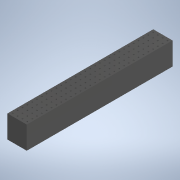
# Autodesk Inventor part: PCIconnector
Saved by Autodesk Inventor 2022 (Build 260153000, 153)
## iProperties
Created: 2021-10-06
Part Number: PCIconnector
Material: Generic
Document SubType Name: Modeling
Designer: Bowen O'Steen
Density: 1 g/cm^3
Appearance: Dark Gray
Author: Bowen O'Steen
Autodesk Inventor part; units mm, degrees
ref_plane "YZ Plane" through (0, 0, 0) normal (1, 0, 0) x (0, 1, 0)
ref_plane "XZ Plane" through (0, 0, 0) normal (0, 1, 0) x (-1, 0, 0)
ref_plane "XY Plane" through (0, 0, 0) normal (0, 0, 1) x (1, 0, 0)
sketch "Sketch1" plane through (0, 0, 0) normal (0, 1, 0) x (-1, 0, 0)
  line L0 (4, 30.15) -> (-4, 30.15)
  line L1 (-4, 30.15) -> (-4, -30.15)
  line L2 (-4, -30.15) -> (4, -30.15)
  line L3 (4, -30.15) -> (4, 30.15)
  point P0 (0, 0)
  point P1 (4, 0)
  point P2 (0, -30.15)
  dimension "d0" = 8
  dimension "d1" = 60.3
  constraints: 8 end point, 2 midpoint, 2 parallel, 1 horizontal, 1 horizontal alignment, 1 perpendicular, 1 vertical alignment
  measures "d0" distance of L1.end L2.end
  measures "d1" distance of L2.end L0.start
extrude "Extrusion1" add sketch "Sketch1" along normal blind 9.35
sketch "Sketch2" plane through (0, 9.35, 0) normal (0, 1, 0) x (1, 0, 0)
  line L0 (-3.25, 28.75) -> (-2.75, 28.75)
  line L1 (-2.75, 28.75) -> (-2.75, 29.25)
  line L2 (-2.75, 29.25) -> (-3.25, 29.25)
  line L3 (-3.25, 29.25) -> (-3.25, 28.75)
  line L4 (-4, 30.15) -> (-4, -30.15) projected
  line L5 (4, 30.15) -> (-4, 30.15) projected
  point P0 (0, 0)
  dimension "d4" = 0.5
  dimension "d5" = 0.5
  dimension "d6" = 0.75
  dimension "d7" = 0.9
  constraints: 8 end point, 2 parallel, 1 horizontal, 1 perpendicular
  measures "d4" distance of L2.end L0.start
  measures "d5" distance of L1.end L2.end
  measures "d6" distance between parallel lines of L4 L3
  measures "d7" distance between parallel lines of L5 L2
extrude "Extrusion2" cut sketch "Sketch2" against normal through all
pattern_linear "Rectangular Pattern1" count 30 spacing 2 along (0, 0, 1) count 4 spacing 2 along (1, 0, 0) of "Extrusion2"
equation "\"d5\" = d4"
body "Solid1"
